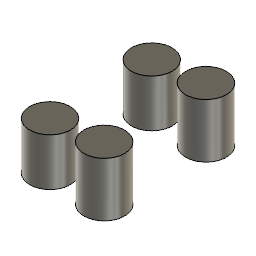
player_card (Autodesk Fusion 360 archive; units mm, degrees)
design "cap"
part number: 2026-05-19-05-25-21-859
Autodesk Fusion 360 part; units mm, degrees
other "DerivedContext1"
other "DerivedContext2"
sketch "sketch 280" plane through (0, 0, 0) normal (0, 0, 1) x (1, 0, 0)
  line L0 (49.5649, -39.1107) -> (119.2642, -39.1107)
  line L1 (119.2642, -39.1107) -> (119.2642, -158.8963)
  line L2 (119.2642, -158.8963) -> (49.5649, -158.8963)
  line L3 (49.5649, -158.8963) -> (49.5649, -39.1107)
  line L4 (121.7642, -161.3963) -> (47.0649, -161.3963)
  line L5 (47.0649, -161.3963) -> (47.0649, -36.6107)
  line L6 (47.0649, -36.6107) -> (121.7642, -36.6107)
  line L7 (121.7642, -36.6107) -> (121.7642, -161.3963)
  line L8 (68, -84) -> (101.7549, -84)
  line L9 (101.7549, -84) -> (101.7549, -53.4795)
  line L10 (101.7549, -53.4795) -> (68, -53.4795)
  line L11 (68, -53.4795) -> (68, -84)
  line L12 (67.5, -84.5) -> (102.2549, -84.5)
  line L13 (102.2549, -84.5) -> (102.2549, -52.9795)
  line L14 (102.2549, -52.9795) -> (67.5, -52.9795)
  line L15 (67.5, -52.9795) -> (67.5, -84.5)
  circle A0 centre (102, -125) radius 3.25
  circle A1 centre (67, -125) radius 3.25
  circle A2 centre (84.4762, -125) radius 3.25
  circle A3 centre (84.4762, -109.2563) radius 3.25
  circle A4 centre (84.4762, -141.496) radius 3.25
  circle A5 centre (112, -152) radius 0.9
  circle A6 centre (112, -152) radius 2.4
  circle A7 centre (111.993, -46.5018) radius 0.9
  circle A8 centre (111.993, -46.5018) radius 2.4
  circle A9 centre (55.4694, -102.876) radius 2.4
  circle A10 centre (55.4694, -102.876) radius 0.9
  line L16 (120.7642, -160.3963) -> (48.0649, -160.3963)
  line L17 (48.0649, -160.3963) -> (48.0649, -37.6107)
  line L18 (48.0649, -37.6107) -> (120.7642, -37.6107)
  line L19 (120.7642, -37.6107) -> (120.7642, -160.3963)
  circle A11 centre (8.6805, -81.9068) radius 1.65
  circle A12 centre (8.6805, -81.9068) radius 3
  line L20 (92.7082, -95.8162) -> (63.7082, -95.8162) construction
  line L21 (63.7082, -95.8162) -> (63.7082, -82.8162) construction
  line L22 (63.7082, -82.8162) -> (92.7082, -82.8162) construction
  line L23 (92.7082, -82.8162) -> (92.7082, -95.8162) construction
  circle A13 centre (8.6805, -81.9068) radius 1.65
  circle A14 centre (8.6805, -81.9068) radius 3
  circle A15 centre (8.6805, -96.9068) radius 3
  circle A16 centre (8.6805, -96.9068) radius 3
  circle A17 centre (8.6805, -96.9068) radius 1.7
extrude "拉伸1" add sketch "sketch 280" along normal blind 9 contours A12 A14 makes body 1
extrude "拉伸2" add sketch "sketch 280" against normal blind 0.5 from surface at 9 contours A11 A13 bodies 1
move_body "移动1" bodies 1 to x (1, 0, 0) y (0, 1, 0) z (0, 0, 1) at (93.3, -8.1, 11)
move_body "移动2" bodies 1 to x (1, 0, 0) y (0, 1, 0) z (0, 0, 1) at (0, 0, 14)
extrude "拉伸3" add 1 faces at (104.3326, -90.9741, 25) along direction (0, 0, -1) blind 4 on bodies 1 bodies 1
move_body "移动3" bodies 1 to x (1, 0, 0) y (0, 1, 0) z (0, 0, 1) at (0, 0, -3)
move_body "移动4" bodies 1 to x (1, 0, 0) y (0, 1, 0) z (0, 0, 1) at (0, 0, 4)
extrude "拉伸4" cut 1 faces at (104.3326, -90.9741, 22) along direction (0, 0, 1) blind 3 on bodies 1 bodies 1
extrude "拉伸5" cut 1 faces at (104.3326, -90.9741, 25) along direction (0, 0, 1) blind 2 on bodies 1 bodies 1
copy_body "复制和粘贴实体1" bodies 1 makes body 2
move_body "移动5" bodies 2 to x (1, 0, 0) y (0, 1, 0) z (0, 0, 1) at (0, -9, 0)
move_body "移动6" bodies 1 to x (1, 0, 0) y (0, 1, 0) z (0, 0, 1) at (0, 3, 0)
sketch "草图1" plane through (0, 0, 0) normal (0, 0, 1) x (1, 0, 0)
copy_body "复制和粘贴实体2" bodies 1 makes body 3
move_body "移动7" bodies 3 to x (1, 0, 0) y (0, 1, 0) z (0, 0, 1) at (0, 11, 0)
extrude "拉伸6" add 1 faces at (104.3326, -99.9741, 27) along direction (0, 0, -1) blind 1 on bodies 2 bodies 2
extrude "拉伸7" cut 1 faces at (104.3326, -76.9741, 27) along direction (0, 0, 1) blind 1 on bodies 3 bodies 3
sketch "sketch 1258" plane through (0, 0, 0) normal (0, 0, 1) x (1, 0, 0)
  line L0 (49.5649, -39.1107) -> (119.2642, -39.1107)
  line L1 (119.2642, -39.1107) -> (119.2642, -158.8963)
  line L2 (119.2642, -158.8963) -> (49.5649, -158.8963)
  line L3 (49.5649, -158.8963) -> (49.5649, -39.1107)
  line L4 (121.7642, -161.3963) -> (47.0649, -161.3963)
  line L5 (47.0649, -161.3963) -> (47.0649, -36.6107)
  line L6 (47.0649, -36.6107) -> (121.7642, -36.6107)
  line L7 (121.7642, -36.6107) -> (121.7642, -161.3963)
  line L8 (68, -84) -> (101.7549, -84)
  line L9 (101.7549, -84) -> (101.7549, -53.4795)
  line L10 (101.7549, -53.4795) -> (68, -53.4795)
  line L11 (68, -53.4795) -> (68, -84)
  line L12 (67.5, -84.5) -> (102.2549, -84.5)
  line L13 (102.2549, -84.5) -> (102.2549, -52.9795)
  line L14 (102.2549, -52.9795) -> (67.5, -52.9795)
  line L15 (67.5, -52.9795) -> (67.5, -84.5)
  circle A0 centre (102, -125) radius 3.25
  circle A1 centre (67, -125) radius 3.25
  circle A2 centre (84.4762, -125) radius 3.25
  circle A3 centre (84.4762, -109.2563) radius 3.25
  circle A4 centre (84.4762, -141.496) radius 3.25
  circle A5 centre (112, -152) radius 0.9
  circle A6 centre (112, -152) radius 2.4
  circle A7 centre (111.993, -46.5018) radius 0.9
  circle A8 centre (111.993, -46.5018) radius 2.4
  circle A9 centre (55.4694, -102.876) radius 2.4
  circle A10 centre (55.4694, -102.876) radius 0.9
  line L16 (120.7642, -160.3963) -> (48.0649, -160.3963)
  line L17 (48.0649, -160.3963) -> (48.0649, -37.6107)
  line L18 (48.0649, -37.6107) -> (120.7642, -37.6107)
  line L19 (120.7642, -37.6107) -> (120.7642, -160.3963)
  circle A11 centre (8.6805, -81.9068) radius 1.65
  circle A12 centre (8.6805, -81.9068) radius 3
  line L20 (92.7082, -95.8162) -> (63.7082, -95.8162) construction
  line L21 (63.7082, -95.8162) -> (63.7082, -82.8162) construction
  line L22 (63.7082, -82.8162) -> (92.7082, -82.8162) construction
  line L23 (92.7082, -82.8162) -> (92.7082, -95.8162) construction
  circle A13 centre (8.6805, -81.9068) radius 1.65
  circle A14 centre (8.6805, -81.9068) radius 3
  circle A15 centre (8.6805, -96.9068) radius 3
  circle A16 centre (8.6805, -96.9068) radius 3
  circle A17 centre (8.6805, -96.9068) radius 1.7
extrude "拉伸8" add sketch "sketch 1258" along normal blind 7 separate body contours A12 A14 makes body 4
extrude "拉伸9" add sketch "sketch 1258" against normal blind 0.5 from surface at 7 contours A11 A13 bodies 4
copy_body "复制和粘贴实体3" bodies 4 makes body 5
move_body "移动8" bodies 5 to x (1, 0, 0) y (0, 1, 0) z (0, 0, 1) at (8, 0, 0)
extrude "拉伸10" add 1 faces at (16.458, -80.9319, 7) along direction (0, 0, 1) blind 1 on bodies 5 bodies 5
extrude "拉伸11" cut 1 faces at (16.5581, -81.3706, 6.5) along direction (0, 0, 1) blind 1 on bodies 5 bodies 5
extrude "拉伸12" add sketch "sketch 1258" along normal blind 7 separate body contours A15 A16 makes body 6
extrude "拉伸13" add sketch "sketch 1258" against normal blind 0.5 from surface at 7 contours A17 bodies 6
copy_body "复制和粘贴实体4" bodies 6 makes body 7
move_body "移动9" bodies 7 to x (1, 0, 0) y (0, 1, 0) z (0, 0, 1) at (8, 0, 0)
extrude "拉伸14" add 1 faces at (16.458, -95.9319, 7) along direction (0, 0, 1) blind 1 on bodies 7 bodies 7
extrude "拉伸15" cut 1 faces at (16.3888, -97.4343, 6.5) along direction (0, 0, 1) blind 1 on bodies 7 bodies 7
hidden bodies 1 2 3
